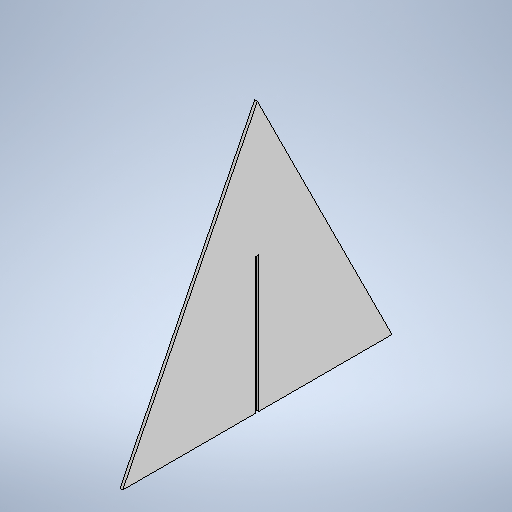
# Autodesk Inventor part: MSC 207 CONE BLADE
Saved by Autodesk Inventor 2025 (Build 290162010, 162A)
## iProperties
Created: 2025-01-15
Part Number: MSC 207 CONE BLADE
Material: Stainless Steel
Document SubType Name: Sheet Metal
Designer: pokla
Density: 8 g/cm^3
Sheet Metal Rule: AISI304 3mm Die 32
Appearance: Default
Author: pokla
Autodesk Inventor part; units mm, degrees
ref_plane "YZ Plane" through (0, 0, 0) normal (1, 0, 0) x (0, 1, 0)
ref_plane "XZ Plane" through (0, 0, 0) normal (0, 1, 0) x (-1, 0, 0)
ref_plane "XY Plane" through (0, 0, 0) normal (0, 0, 1) x (1, 0, 0)
sketch "Sketch1" plane through (0, 0, 0) normal (1, 0, 0) x (0, 1, 0)
  line L0 (150, 0) -> (-150, 0)
  line L1 (0, 0) -> (0, 300)
  line L2 (0, 300) -> (150, 0)
  line L3 (0, 300) -> (-150, 0)
  dimension "d0" = 300
  dimension "d1" = 300
  measures "d0" distance of L0.start L0.end
  measures "d1" distance of L1.start L1.end
extrude "Plate1" add sketch "Sketch1" along normal mid plane 3
sketch "Sketch3" plane through (1.5, 0, 0) normal (1, 0, 0) x (0, 0, -1)
  line L0 (0, -1.6) -> (-151, -1.6)
  line L1 (-151, -1.6) -> (-151, 1.6)
  line L2 (-151, 1.6) -> (0, 1.6)
  line L3 (0, 1.6) -> (0, -1.6)
  line L4 (0, 150) -> (0, -150) projected
  point P0 (0, 0)
  point P1 (0, 0)
  dimension "d7" = 3.2
  dimension "d8" = 151
  constraints: 8 end point, 2 midpoint, 2 parallel, 1 horizontal, 1 perpendicular
  measures "d7" distance of L2.end L0.start
  measures "d8" distance between parallel lines of L3 L1
extrude "Extrusion2" cut sketch "Sketch3" against normal through all
equation "\"d2\" = Thickness"
equation "\"BendReliefWidth\" = Thickness"
equation "\"BendReliefDepth\" = 0.5 * Thickness"
equation "\"CornerReliefSize\" = 4 * Thickness"
equation "\"MinimumRemnant\" = 2 * Thickness"
equation "\"TransitionRadius\" = BendRadius"
equation "\"JacobiRadiusSize\" = BendRadius"
equation "\"GapSize\" = Thickness"
equation "\"Thickness\" = 3"
equation "\"BendRadius\" = 5"
body "Solid1"
